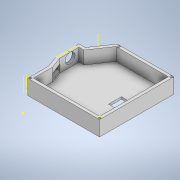
# Autodesk Inventor part: Case
Saved by Autodesk Inventor 2020.1 (Build 241239000, 239)
## iProperties
Created: 2020-05-23
Part Number: Case
Material: Generic
Document SubType Name: Modeling
Designer: super
Density: 1 g/cm^3
Appearance: Default
Author: super
Autodesk Inventor part; units mm, degrees
ref_plane "YZ Plane" through (0, 0, 0) normal (1, 0, 0) x (0, 1, 0)
ref_plane "XZ Plane" through (0, 0, 0) normal (0, 1, 0) x (-1, 0, 0)
ref_plane "XY Plane" through (0, 0, 0) normal (0, 0, 1) x (1, 0, 0)
sketch "Sketch1" plane through (0, 0, 0) normal (0, 1, 0) x (-1, 0, 0)
  line L0 (0, 0) -> (49.1, 0)
  line L1 (49.1, -47.9) -> (0, -47.9)
  line L2 (0, -47.9) -> (0, 0)
  line L3 (46.7, -10.9) -> (49.1, -18.9)
  line L4 (46.7, -10.9) -> (46.7, 0)
  line L5 (49.1, 0) -> (46.7, 0)
  line L6 (49.1, -18.9) -> (49.1, -47.9)
  dimension "d0" = 49.1
  dimension "d1" = 47.9
  dimension "d2" = 18.9
  constraints: 14 end point, 1 collinear, 1 horizontal, 1 parallel, 1 perpendicular, 1 point on line
  measures "d0" distance of L1.start L1.end
  measures "d1" distance of L0.end L1.start
  measures "d2" distance of L0.end L3.end
extrude "Extrusion1" add sketch "Sketch1" along normal blind 1.5
sketch "Sketch2" plane through (0, 1.5, 0) normal (0, 1, 0) x (1, 0, 0)
  line L0 (-49.1, 18.9) -> (-46.7, 10.9) projected
  line L1 (-46.2, 10.9) -> (-46.2, 0)
  line L2 (-46.2, 0) -> (-46.7, 0)
  line L3 (-46.7, 10.9) -> (-46.7, 0) projected
  line L4 (-46.7, 0) -> (-46.7, 10.9)
  line L5 (-49.1, 47.9) -> (-49.1, 18.9) projected
  line L6 (-46.7, 10.9) -> (-49.1, 18.9)
  line L7 (-49.1, 18.9) -> (-46.2, 10.9)
  point P0 (0, 0)
  constraints: 10 end point, 1 collinear, 1 perpendicular
extrude "Extrusion2" cut sketch "Sketch2" against normal blind 10
sketch "Sketch3" plane through (0, 1.5, 0) normal (0, 1, 0) x (1, 0, 0)
  line L0 (-49.1, 47.9) -> (-49.1, 18.9) projected
  line L1 (-49.1, 34.5784) -> (-45.5979, 34.5784)
  line L2 (-45.5979, 34.5784) -> (-36.4784, 47.9)
  line L3 (0, 47.9) -> (-49.1, 47.9) projected
  line L4 (-49.1, 47.9) -> (-36.4784, 47.9)
  line L5 (-49.1, 47.9) -> (-49.1, 34.5784)
  point P0 (0, 0)
  constraints: 8 end point, 2 point on line, 1 horizontal, 1 parallel, 1 perpendicular
extrude "Extrusion3" cut sketch "Sketch3" against normal blind 10
sketch "Sketch4" plane through (0, 1.5, 0) normal (0, 1, 0) x (1, 0, 0)
  line L0 (-46.2, 10.9) -> (-49.1, 18.9) projected
  line L1 (-46.2, 0) -> (0, 0) projected
  line L2 (-46.2, -2) -> (0, -2)
  line L3 (0, -2) -> (2, -2)
  line L4 (2, -2) -> (2, 47.9)
  line L5 (0, 47.9) -> (-36.4784, 47.9) projected
  line L6 (2, 47.9) -> (2, 49.9)
  line L7 (2, 49.9) -> (-36.4784, 49.9)
  line L8 (-38.1287, 49.0298) -> (-37.533, 49.9)
  line L9 (-37.533, 49.9) -> (-36.4784, 49.9)
  line L10 (-45.5979, 34.5784) -> (-36.4784, 47.9) projected
  line L11 (-49.1, 36.5784) -> (-46.6525, 36.5784)
  line L12 (-46.6525, 36.5784) -> (-37.533, 49.9)
  line L13 (-46.2, -2) -> (-48.2, -2)
  line L14 (-48.2, -2) -> (-48.2, 10.9)
  line L15 (-51.1, 18.9) -> (-48.2, 10.9)
  line L16 (-49.1, 36.5784) -> (-51.1, 36.5784)
  line L17 (-51.1, 36.5784) -> (-51.1, 18.9)
  line L18 (0, 0) -> (0, 47.9) projected
  line L19 (0, 0) -> (0, 47.9)
  line L20 (0, 47.9) -> (-36.4784, 47.9)
  line L21 (-36.4784, 47.9) -> (-45.5979, 34.5784)
  line L22 (-45.5979, 34.5784) -> (-49.1, 34.5784) projected
  line L23 (-49.1, 34.5784) -> (-45.5979, 34.5784)
  line L24 (-49.1, 34.5784) -> (-49.1, 18.9) projected
  line L25 (-49.1, 34.5784) -> (-49.1, 18.9)
  line L26 (-49.1, 18.9) -> (-46.2, 10.9)
  line L27 (-46.2, 0) -> (-46.2, 10.9)
  line L28 (-46.2, 0) -> (0, 0)
  dimension "d16" = 2
  dimension "d17" = 2
  dimension "d18" = 2
  dimension "d23" = 2
  constraints: 44 end point, 4 collinear, 4 horizontal, 4 perpendicular, 3 point on line, 2 vertical
  measures "d16" distance of L1.start L2.start
  measures "d17" distance of L2.end L3.end
  measures "d18" distance of L4.end L6.end
  measures "d23" distance of L2.start L13.end
extrude "Extrusion4" add sketch "Sketch4" along normal blind 9
sketch "Sketch5" plane through (0, 0, 0) normal (0, -1, 0) x (1, 0, 0)
  line L0 (-46.2, 0) -> (0, 0) projected
  line L1 (0, 0) -> (-46.2, 0)
  line L2 (-46.2, 0) -> (-46.2, -10.9) projected
  line L3 (-46.2, 0) -> (-46.2, -10.9)
  line L4 (-46.2, -10.9) -> (-49.1, -18.9) projected
  line L5 (-46.2, -10.9) -> (-49.1, -18.9)
  line L6 (-49.1, -18.9) -> (-49.1, -34.5784) projected
  line L7 (-49.1, -18.9) -> (-49.1, -34.5784)
  line L8 (-49.1, -34.5784) -> (-45.5979, -34.5784) projected
  line L9 (-49.1, -34.5784) -> (-45.5979, -34.5784)
  line L10 (-36.4784, -47.9) -> (-45.5979, -34.5784) projected
  line L11 (-45.5979, -34.5784) -> (-36.4784, -47.9)
  line L12 (-36.4784, -47.9) -> (0, -47.9) projected
  line L13 (-36.4784, -47.9) -> (0, -47.9)
  line L14 (0, -47.9) -> (0, 0)
  line L15 (-48.2, 2) -> (2, 2) projected
  line L16 (2, 2) -> (-48.2, 2)
  line L17 (-51.1, -18.9) -> (-48.2, -10.9) projected
  line L18 (-48.2, 2) -> (-48.2, -10.9)
  line L19 (-48.2, -10.9) -> (-51.1, -18.9)
  line L20 (-51.1, -18.9) -> (-51.1, -36.5784)
  line L21 (-46.6525, -36.5784) -> (-51.1, -36.5784) projected
  line L22 (-51.1, -36.5784) -> (-46.6525, -36.5784)
  line L23 (-37.533, -49.9) -> (-46.6525, -36.5784) projected
  line L24 (-46.6525, -36.5784) -> (-37.533, -49.9)
  line L25 (2, 2) -> (2, -49.9) projected
  line L26 (-37.533, -49.9) -> (2, -49.9)
  line L27 (2, -49.9) -> (2, 2)
  constraints: 32 end point, 7 perpendicular, 5 collinear, 3 horizontal, 1 parallel
extrude "Extrusion5" add sketch "Sketch5" against normal blind 1.5
sketch "Sketch6" plane through (0, 10.5, 0) normal (0, 1, 0) x (1, 0, 0)
  line L0 (-48.2, -2) -> (2, -2) projected
  circle A0 centre (1, -1) radius 0.75
  line L1 (-46.2, 0) -> (-46.2, 10.9) projected
  circle A1 centre (-47.2, -1) radius 0.75
  point P0 (0, 0)
  dimension "d35" = 1.5
  constraints: 2 centre point
  measures "d35" diameter of A1
sketch "Sketch7" plane through (0, 10.5, 0) normal (0, 1, 0) x (1, 0, 0)
  point P0 (0, 0)
extrude "Extrusion6" cut sketch "Sketch6" against normal blind 7.5
sketch "Sketch8" plane through (0, 10.5, 0) normal (0, 1, 0) x (1, 0, 0)
  line L0 (-45.5979, 34.5784) -> (-36.4784, 47.9) projected
  circle A0 centre (-35.4784, 48.9) radius 0.75
  circle A1 centre (1, 48.9) radius 0.75
  point P0 (0, 0)
  dimension "d40" = 1.5
  dimension "d43" = 1.5
  constraints: 2 centre point
  measures "d40" diameter of A0
  measures "d43" diameter of A1
extrude "Extrusion7" cut sketch "Sketch8" against normal blind 7.5
sketch "Sketch9" plane through (0, 0, 0) normal (0, -1, 0) x (1, 0, 0)
  line L0 (-48.2, 2) -> (2, 2) projected
  line L1 (2, 2) -> (2, -49.9) projected
  line L2 (-6.75, -23.95) -> (-6.75, -19.45)
  line L3 (-6.75, -19.45) -> (-13.25, -19.45)
  line L4 (-13.25, -19.45) -> (-13.25, -28.45)
  line L5 (-13.25, -28.45) -> (-6.75, -28.45)
  line L6 (-6.75, -28.45) -> (-6.75, -23.95)
  point P0 (0, 0)
  dimension "d51" = 6.5
  dimension "d52" = 9
  constraints: 10 end point, 4 perpendicular, 1 point on line
  measures "d51" distance of L2.end L3.end
  measures "d52" distance of L3.end L4.end
extrude "Extrusion8" cut sketch "Sketch9" against normal blind 1.5
sketch "Sketch10" plane through (0, 10.5, 0) normal (0, 1, 0) x (1, 0, 0)
  line L0 (-49.1, 18.9) -> (-46.2, 10.9) projected
  line L1 (-48.2, -2) -> (-48.2, 10.9) projected
  line L2 (-48.2, 10.9) -> (-51.1, 18.9) projected
  line L3 (-48.2, 10.175) -> (-48.2, 10.9)
  line L4 (-51.1, 18.9) -> (-51.1, 36.5784) projected
  line L5 (-51.1, 18.175) -> (-51.1, 18.9)
  line L6 (-51.1, 18.175) -> (-48.2, 10.175)
  line L7 (-48.2, 10.9) -> (-51.1, 18.9)
  point P0 (0, 0)
  constraints: 8 end point, 2 collinear, 1 parallel, 1 point on line
extrude "Extrusion9" add sketch "Sketch10" against normal blind 10.5
sketch "Sketch11" plane through (-51.1, 0, -18.175) normal (-0.9401361, 0, 0.3407993) x (0.3407993, 0, 0.9401361)
  point P0 (34.5018, 0)
sketch "Sketch12" plane through (-51.1, 0, -18.175) normal (-0.9401361, 0, 0.3407993) x (0.3407993, 0, 0.9401361)
  line L0 (0, 10.5) -> (0, 0) projected
  line L1 (5.4546, 0) -> (3.2394, 0) projected
  line L2 (4.2545, 0) -> (7.2545, 0) construction
  line L3 (4.2545, 7) -> (0, 7)
  line L4 (0, 7) -> (0, 3)
  line L5 (0, 3) -> (8.5094, 3)
  line L6 (8.5094, 1.5) -> (8.5094, 10.5) projected
  line L7 (4.2545, 7) -> (8.5094, 7)
  line L8 (8.5094, 10.5) -> (8.5094, 0) projected
  line L9 (8.5094, 3) -> (8.5094, 7)
  line L10 (0, 10.5) -> (8.5094, 10.5) projected
  line L11 (0, 10.5) -> (0, 0) projected
  line L12 (8.5094, 0) -> (0, 0) projected
  line L13 (8.5094, 10.5) -> (8.5094, 0) projected
  point P0 (34.5018, 0)
  dimension "d58" = 4.2545
  constraints: 12 end point, 5 point on line, 3 perpendicular, 1 horizontal
  measures "d58" distance of L0.end L2.start
extrude "Extrusion10" cut sketch "Sketch12" along normal blind 5 contours L3 L7 L6 L5 L0
sketch "Sketch14" plane through (0, 10.5, 0) normal (0, 1, 0) x (1, 0, 0)
  point P0 (0, 0)
sketch "Sketch15" plane through (0, 10.5, 0) normal (0, 1, 0) x (1, 0, 0)
  line L0 (-46.2, 0) -> (-46.2, 10.9) projected
  line L1 (-46.2, 10.9) -> (-46.2, 11.9)
  line L2 (-46.2, 11.9) -> (-49.1, 19.8981)
  line L3 (-49.1, 34.5784) -> (-49.1, 18.9) projected
  line L4 (-46.2, 11.9) -> (-37.6924, 11.9) construction
  line L5 (-49.1, 19.8981) -> (-49.1, 18.9)
  line L6 (-49.1, 18.9) -> (-46.2, 10.9) projected
  line L7 (-49.1, 18.9) -> (-46.2, 10.9)
  point P0 (0, 0)
  dimension "d71" = 1
  dimension "d72" = 109.93
  constraints: 10 end point, 1 collinear, 1 equal length, 1 horizontal, 1 point on line, 1 vertical
  measures "d71" distance of L0.end L1.end
  measures "d72" angle of L4 L2
extrude "Extrusion12" add sketch "Sketch15" against normal blind 9
sketch "Sketch16" plane through (0, 10.5, 0) normal (0, 1, 0) x (1, 0, 0)
  line L0 (-51.1, 18.175) -> (-48.2, 10.175) projected
  line L1 (-51.1, 18.175) -> (-51.1, 19.175)
  line L2 (-51.1, 36.5784) -> (-51.1, 18.175) projected
  line L3 (-51.1, 19.175) -> (-48.2, 11.1769)
  line L4 (-51.1, 19.175) -> (-42.5924, 19.175) construction
  line L5 (-48.2, 11.1769) -> (-48.2, 10.175)
  line L6 (-48.2, 10.175) -> (-48.2, -2) projected
  line L7 (-51.1, 18.175) -> (-48.2, 10.175)
  point P0 (0, 0)
  dimension "d75" = 1
  dimension "d76" = 70.07
  constraints: 10 end point, 1 equal length, 1 horizontal, 1 point on line, 1 vertical
  measures "d75" distance of L0.start L1.end
  measures "d76" angle of L3 L4
extrude "Extrusion13" cut sketch "Sketch16" against normal blind 10.5
sketch "Sketch17" plane through (-51.1, 0, -36.5784) normal (-1, 0, 0) x (0, 0, 1)
  line L0 (-13.3216, 0) -> (-13.3216, 10.5) projected
  line L1 (36.8284, 10.5) -> (36.8284, 3) projected
  line L2 (38.5784, 0) -> (38.5784, 10.5) projected
  line L3 (15.9784, 5.25) -> (15.9784, 10.5) construction
  line L4 (16.6804, 10.5) -> (2, 10.5) projected
  point P0 (36.5784, 0)
  constraints: 2 end point, 1 point on line
sketch "Sketch18" plane through (0, 10.5, 0) normal (0, 1, 0) x (1, 0, 0)
  line L0 (-51.1, 19.175) -> (-51.1, 36.5784) projected
  line L1 (-51.1, 19.175) -> (-51.1, 20.6)
  line L2 (-51.1, 20.6) -> (-48.2, 12.6019)
  line L3 (-51.1, 20.6) -> (-42.5924, 20.6) construction
  line L4 (-51.1, 19.175) -> (-48.2, 11.1769) projected
  line L5 (-48.2, 12.6019) -> (-48.2, 11.1769)
  line L6 (-51.1, 19.175) -> (-48.2, 11.1769)
  point P0 (0, 0)
  dimension "d82" = 1.425
  dimension "d83" = 70.07
  constraints: 10 end point, 1 collinear, 1 equal length, 1 horizontal, 1 point on line, 1 vertical
  measures "d82" distance of L0.start L1.end
  measures "d83" angle of L2 L3
extrude "Extrusion14" cut sketch "Sketch18" against normal blind 10.5
sketch "Sketch19" plane through (0, 10.5, 0) normal (0, 1, 0) x (1, 0, 0)
  line L0 (-46.2, 11.9) -> (-49.1, 19.8981) projected
  line L1 (-46.2, 11.9) -> (-46.2, 13.325)
  line L2 (-46.2, 13.325) -> (-49.1, 21.3231)
  line L3 (-49.1, 19.8981) -> (-49.1, 34.5784) projected
  line L4 (-49.1, 21.3231) -> (-49.1, 19.8981)
  line L5 (-49.1, 19.8981) -> (-46.2, 11.9)
  point P0 (0, 0)
  dimension "d86" = 1.425
  dimension "d87" = 160.07
  constraints: 8 end point, 1 parallel, 1 point on line, 1 vertical
  measures "d86" distance of L0.start L1.end
  measures "d87" angle of L2 L1
extrude "Extrusion15" add sketch "Sketch19" against normal blind 9
sketch "Sketch20" plane through (-51.1, 0, -20.6) normal (-0.9401098, 0, 0.3408718) x (0.3408718, 0, 0.9401098)
  line L0 (0, 3) -> (8.5096, 3)
  line L1 (8.5096, 10.5) -> (8.5096, 1.5) projected
  line L2 (8.5096, 3) -> (8.5096, 7)
  line L3 (8.5096, 7) -> (0.002, 7)
  line L4 (0.002, 10.5) -> (0.002, 1.5) projected
  line L5 (0, 3) -> (0.002, 7)
  point P0 (36.7848, 0)
  point P1 (0, 0)
  point P2 (8.5096, 7)
  dimension "d90" = 3
  dimension "d91" = 4
  constraints: 8 end point, 2 perpendicular, 2 point on line
  measures "d90" distance of point (0, 0) L0.start
  measures "d91" distance of L0.end L2.end
extrude "Extrusion16" cut sketch "Sketch20" against normal blind 10
sketch "Sketch21" plane through (-51.1, 0, -36.5784) normal (-1, 0, 0) x (0, 0, 1)
  point P0 (36.5784, 0)
sketch "Sketch22" plane through (-51.1, 0, -36.5784) normal (-1, 0, 0) x (0, 0, 1)
  line L0 (15.9784, 0) -> (0, 0) projected
  line L1 (17.1284, 0) -> (8.1284, 0) projected
  circle A0 centre (8.1284, 7) radius 3.5
  point P0 (36.5784, 0)
  dimension "d98" = 7
  constraints: 1 centre point
  measures "d98" diameter of A0
extrude "Extrusion17" cut sketch "Sketch22" against normal blind 10
body "Solid1"
